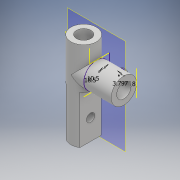
# Autodesk Inventor part: chassiswithdowel
Saved by Autodesk Inventor 2018 (Build 220112000, 112)
## iProperties
Created: 2018-11-04
Part Number: chassiswithdowel
Material: Generic
Document SubType Name: Modeling
Designer: Prakash
Density: 1 g/cm^3
Appearance: Default
Author: Prakash
Autodesk Inventor part; units mm, degrees
ref_plane "YZ Plane" through (0, 0, 0) normal (1, 0, 0) x (0, 1, 0)
ref_plane "XZ Plane" through (0, 0, 0) normal (0, 1, 0) x (-1, 0, 0)
ref_plane "XY Plane" through (0, 0, 0) normal (0, 0, 1) x (1, 0, 0)
sketch "Sketch1" plane through (0, 0, 0) normal (0, 0, 1) x (1, 0, 0)
  line L0 (0, 0) -> (14, 0)
  arc A0 (14, 0) -> (24.3078, 0) centre (19.1539, 1) ccw
  line L1 (24.3078, 0) -> (38.3078, 0)
  line L2 (19.1539, 0) -> (19.1539, 1) construction
  line L3 (14, 0) -> (19.1539, 0) construction
  line L4 (24.3078, 0) -> (19.1539, 0) construction
  line L5 (0, 0) -> (0, -4)
  arc A1 (11.3717, -4) -> (26.9361, -4) centre (19.1539, 1) ccw
  line L6 (0, -4) -> (11.3717, -4)
  line L7 (38.3078, 0) -> (38.3078, -4)
  line L8 (38.3078, -4) -> (26.9361, -4)
  dimension "d0" = 14
  dimension "d2" = 10.5
  dimension "d3" = 14
  dimension "d4" = 1
  dimension "d6" = 4
  dimension "d7" = 18.5
  dimension "d8" = 4
  constraints: 18 end point, 4 horizontal, 4 point on circle, 3 collinear, 3 vertical, 2 centre point, 1 coincident
  measures "d0" distance of L0.start L0.end
  measures "d2" diameter of A0
  measures "d3" distance of L1.start L1.end
  measures "d4" distance of L2.start L2.end
  measures "d6" distance of L0.start L5.end
  measures "d7" diameter of A1
  measures "d8" distance of L1.end L7.end
extrude "Extrusion1" add sketch "Sketch1" along normal blind 10
sketch "Sketch2" plane through (0, 0, 0) normal (0, 0, -1) x (-1, 0, 0)
  line L0 (0, 0) -> (-14, 0) projected
  arc A0 (-24.3078, 0) -> (-14, 0) centre (-19.1539, 1) ccw projected
  line L1 (-24.3078, 0) -> (-38.3078, 0) projected
  line L2 (-38.3078, 0) -> (-38.3078, -4) projected
  line L3 (-38.3078, -4) -> (-26.9361, -4) projected
  arc A1 (-26.9361, -4) -> (-11.3717, -4) centre (-19.1539, 1) ccw projected
  line L4 (-11.3717, -4) -> (0, -4) projected
  line L5 (0, -4) -> (0, 0) projected
  circle A2 centre (-19.1539, 1) radius 5.25
  circle A3 centre (-19.1539, 1) radius 9.25
  dimension "d11" = 4
  constraints: 2 centre point, 2 coincident, 1 concentric
  measures "d11" radial gap between concentric circles of A3 A2
extrude "Extrusion2" add sketch "Sketch2" along normal blind 18.5 contours A3 A1 L1 A0 L0 | L0 A2 L1 A3
ref_plane "Work Plane1" through (28.4039, 1, 0) normal (1, 0, 0) x (0, 1, 0)
sketch "Sketch3" plane through (28.4039, 1, 0) normal (1, 0, 0) x (0, 1, 0)
  line L0 (-9.25, -18.5) -> (9.25, -18.5) projected
  line L1 (-5, 0) -> (-5, 10) projected
  line L2 (-5, 10) -> (-5, 10) projected
  line L3 (-5, 0) -> (-5, 10) projected
  line L4 (-1, 0) -> (-5, 0) projected
  line L5 (-1, 0) -> (-1, 0) projected
  line L6 (-5, 0) -> (-1, 0) projected
  line L7 (-1, 0) -> (5.25, 0) projected
  line L8 (0, 0) -> (0, -18.5) construction
  line L9 (5.25, -18.5) -> (-5.25, -18.5) projected
  circle A0 centre (0, -9.25) radius 5.25
  circle A1 centre (0, -9.25) radius 9.25
  dimension "d14" = 10.5
  dimension "d15" = 18.5
  constraints: 2 centre point, 2 end point, 2 midpoint, 1 coincident, 1 parallel, 1 point on line
  measures "d14" diameter of A0
  measures "d15" diameter of A1
extrude "Extrusion3" add sketch "Sketch3" against normal up to next
extrude "Extrusion4" add sketch "Sketch3" along normal blind 20
sketch "Sketch6" plane through (19.1539, 1, -18.5) normal (0, 0, -1) x (-1, 0, 0)
  circle A0 centre (0, 0) radius 5.25 projected
  circle A1 centre (0, 0) radius 9.25 projected
  arc A2 (9.1958, -1) -> (-9.25, 0) centre (0, 0) ccw projected
  line L0 (-5, 7.7822) -> (-5, -7.7822)
  arc A3 (-9.25, 0) -> (0, -9.25) centre (0, 0) ccw projected
  line L1 (5, 7.7822) -> (5, -7.7822)
  circle A4 centre (0, 0) radius 9.25 projected
  line L2 (0, 9.25) -> (0, -9.25) construction
  arc A5 (5, 7.7822) -> (-5, 7.7822) centre (0, 0) ccw
  arc A6 (-5, -7.7822) -> (5, -7.7822) centre (0, 0) ccw
  point P0 (19.1539, -1)
  dimension "d24" = 10
  constraints: 6 end point, 6 point on circle, 2 centre point, 2 vertical, 1 coincident, 1 parallel, 4 other
  measures "d24" distance between parallel lines of L1 L0
extrude "Extrusion6" add sketch "Sketch6" along normal blind 35 contours L1 A0 L0 | A0 L0 A1 L1 | L1 A1 L0 A0
sketch "Sketch8" plane through (14.1539, -0.6008, -18.5) normal (-1, 0, 0) x (0, 0, 1)
  line L0 (0, 0) -> (0, -6.1814) projected
  line L1 (0, 0) -> (0, 3.2016) projected
  line L2 (0, 9.383) -> (0, 3.2016) projected
  line L3 (0, 9.383) -> (-35, 9.383) projected
  line L4 (-35, -6.1814) -> (-35, 9.383) projected
  line L5 (0, -6.1814) -> (-35, -6.1814) projected
  circle A0 centre (9.25, 1.6008) radius 5.25 projected
  circle A1 centre (9.25, 1.6008) radius 9.25 projected
  circle A2 centre (-20, 1.6008) radius 6.875
  line L6 (-20, 1.6008) -> (-20, 9.383) construction
  line L7 (-20, 1.6008) -> (-20, -6.1814) construction
  circle A3 centre (-20, 1.6008) radius 6.125
  circle A4 centre (-20, 1.6008) radius 3
  point P0 (18.5, 0.6008)
  dimension "d27" = 13.75
  dimension "d28" = 29.25
  dimension "d30" = 12.25
  dimension "d35" = 6
  constraints: 4 end point, 3 centre point, 3 point on line, 2 coincident, 1 collinear, 1 perpendicular
  measures "d27" diameter of A2
  measures "d28" distance of A0.centre L6.start
  measures "d30" diameter of A3
  measures "d35" diameter of A4
extrude "Extrusion7" cut sketch "Sketch8" against normal blind 1 contours A2 | A3 | A4
extrude "Extrusion8" cut sketch "Sketch8" against normal blind 4 contours A3 | A4
extrude "Extrusion9" cut sketch "Sketch8" against normal up to surface (10 mm away) contours A4
ref_plane "Work Plane2" through (28.4039, 10.25, -9.25) normal (0, 1, 0) x (-1, 0, 0)
sketch "Sketch12" plane through (28.4039, 10.25, -9.25) normal (0, 1, 0) x (-1, 0, 0)
  line L0 (-20, 9.25) -> (-20, -9.25) projected
  line L1 (0, 9.25) -> (9.25, 0) projected
  line L2 (9.25, 0) -> (0, 9.25) projected
  line L3 (0, -9.25) -> (9.25, 0) projected
  line L4 (9.25, 0) -> (0, -9.25) projected
  line L5 (0, -9.25) -> (0, 9.25)
  line L6 (0, 0) -> (-20, 0)
  circle A0 centre (-10, 0) radius 4
  point P0 (28.4039, 9.25)
  dimension "d51" = 8
  constraints: 4 end point, 3 midpoint, 1 centre point, 1 vertical
  measures "d51" diameter of A0
extrude "Extrusion11" add sketch "Sketch12" against normal up to surface contours A0 L6 | L6 A0 round surface about axis through (28.4039, 1, -9.25) along (-1, 0, 0) radius 9.25 far side no
extrude "Extrusion12" add sketch "Sketch12" along normal blind 1 contours A0 L6 | L6 A0
sketch "Sketch13" plane through (38.4039, 11.25, -9.25) normal (0, 1, 0) x (1, 0, 0)
  circle A0 centre (0, 0) radius 4 projected
  circle A1 centre (0, 0) radius 2.5275
  point P0 (-38.4039, -9.25)
  dimension "d56" = 5.055
  constraints: 1 centre point, 1 coincident
  measures "d56" diameter of A1
extrude "Extrusion13" cut sketch "Sketch13" against normal blind 3.81 contours A1
sketch "Sketch15" plane through (38.4039, 11.25, -9.25) normal (0, 1, 0) x (1, 0, 0)
  circle A0 centre (0, 0) radius 2.5275 construction
  circle A1 centre (0, 0) radius 4 construction
  circle A2 centre (0, 0) radius 2.6545
  point P0 (-38.4039, -9.25)
  dimension "d60" = 5.309
  constraints: 1 centre point, 1 coincident
  measures "d60" diameter of A2
sketch "Sketch16" plane through (38.4039, 7.44, -9.25) normal (0, 1, 0) x (1, 0, 0)
  circle A0 centre (0, 0) radius 2.5275 projected
  point P0 (-38.4039, -9.25)
loft "Loft1" cut profiles "Sketch15" section 1 edges at (35.8764, 7.44, -9.25)
sketch "Sketch17" plane through (38.4039, 7.44, -9.25) normal (0, 1, 0) x (1, 0, 0)
  circle A0 centre (0, 0) radius 2.5275 construction
  circle A1 centre (0, 0) radius 1.8985
  point P0 (-38.4039, -9.25)
  dimension "d65" = 3.797
  constraints: 1 centre point, 1 coincident
  measures "d65" diameter of A1
sketch "Sketch18" plane through (0, 0, 10) normal (0, 0, 1) x (1, 0, 0)
  line L0 (14, 0) -> (0, 0) projected
  line L1 (0, 0) -> (0, -4) projected
  line L2 (0, -4) -> (11.3717, -4) projected
  arc A0 (11.3717, -4) -> (26.9361, -4) centre (19.1539, 1) ccw projected
  line L3 (26.9361, -4) -> (38.3078, -4) projected
  line L4 (38.3078, -4) -> (38.3078, 0) projected
  line L5 (38.3078, 0) -> (24.3078, 0) projected
  arc A1 (14, 0) -> (24.3078, 0) centre (19.1539, 1) ccw projected
extrude "Extrusion14" cut sketch "Sketch18" against normal up to surface (10 mm away)
sketch "Sketch19" plane through (19.1539, 1, 0) normal (0, 0, 1) x (1, 0, 0)
  circle A0 centre (0, 0) radius 5.25 projected
  circle A1 centre (0, 0) radius 9.25 projected
  point P0 (-19.1539, -1)
  point P1 (9.25, 0)
  constraints: 1 horizontal alignment
extrude "Extrusion15" add sketch "Sketch19" along normal blind 30 from surface at -18.5
body "Solid1"
